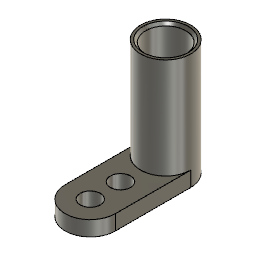
LED strip fixture (Autodesk Fusion 360 design; units mm, degrees)
part number: 2026-05-07-12-59-44-376
Autodesk Fusion 360 part; units mm, degrees
sketch "Sketch1" plane through (0, 0, 0) normal (0, 0, 1) x (1, 0, 0)
  circle A0 centre (0, 0) radius 5
  dimension "d1" = 10
  constraint coincident A0.centre origin
  measures "d1" diameter of A0
extrude "Extrude1" add sketch "Sketch1" along normal blind 20 thin wall 1 inside makes body 1
extrude "Extrude2" add sketch "Sketch1" against normal blind 3 separate body makes body 2
sketch "Sketch2" plane through (0, 0, 0) normal (0, 0, 1) x (1, 0, 0)
  line L0 (-5, -15) -> (-5, 0)
  line L1 (-5, 0) -> (5, 0)
  line L2 (5, 0) -> (5, -15)
  arc A0 (-5, -15) -> (5, -15) centre (0, -15) ccw
  constraint tangent L0 A0
  constraint vertical L0
  constraint perpendicular L0 L1
  constraint tangent L2 A0
  constraint perpendicular L1 L2
extrude "Extrude3" add sketch "Sketch2" against normal blind 3 bodies 1 2
sketch "Sketch3" plane through (0, 0, 0) normal (0, 0, 1) x (1, 0, 0)
  circle A0 centre (0, 0) radius 1.5
  dimension "d10" = 3
  measures "d10" diameter of A0
extrude "Extrude4" cut sketch "Sketch3" against normal blind 3 bodies 1
chamfer "Chamfer1" distance 0.5 angle 45 1 edges at (-3.7293, 1.4465, 20) on bodies 1
sketch "Sketch4" plane through (0, 0, 0) normal (0, 0, 1) x (1, 0, 0)
  circle A0 centre (0, -15) radius 2
  circle A1 centre (0, -9) radius 2
  dimension "d14" = 4
  dimension "d15" = 4
  measures "d14" diameter of A0
  measures "d15" diameter of A1
extrude "Extrude5" cut sketch "Sketch4" against normal blind 3 bodies 1
